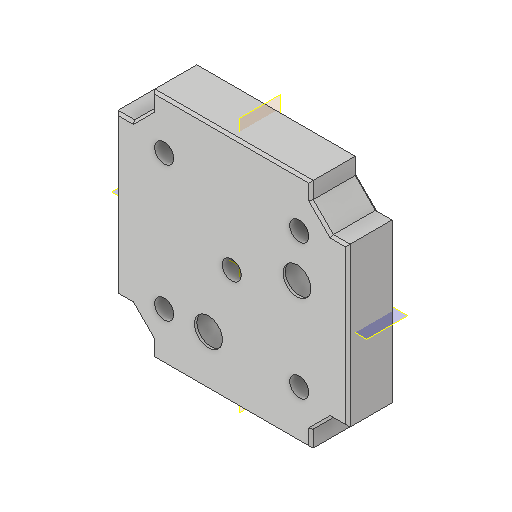
# Autodesk Inventor part: 20_Cube_Insert_Kinematic_Mirror_90_pro_magnetic
Saved by Autodesk Inventor 2022 (Build 260153000, 153)
## iProperties
Created: 2019-07-01
Part Number: 20_Cube_Insert_Kinematic_Mirror_90_pro_magnetic
Material: Generic
Document SubType Name: Modeling
Designer: diederichbenedict
Density: 1 g/cm^3
Appearance: Default
Catalog Web Link: isPrinted
Vendor: openUC2
Author: diederichbenedict
Autodesk Inventor part; units mm, degrees
ref_plane "YZ Plane" through (0, 0, 0) normal (1, 0, 0) x (0, 1, 0)
ref_plane "XZ Plane" through (0, 0, 0) normal (0, 1, 0) x (-1, 0, 0)
ref_plane "Work Plane1" through (0, 0, 10) normal (0, 0, 1) x (1, 0, 0)
sketch "Sketch1" plane through (0, 0, 10) normal (0, 0, 1) x (1, 0, 0)
  line L0 (-4.0299, -0.3538) -> (-2.2322, 1.4439) construction
  arc A0 (-1.4439, 2.2322) -> (-2.2322, 1.4439) centre (-0.9299, 0.9299) ccw construction
  line L1 (-1.4439, 2.2322) -> (0.3538, 4.0299) construction
  line L2 (-37.8299, 42.8299) -> (-37.8299, 37.8299) construction
  line L3 (-37.8299, 37.8299) -> (-42.9208, 37.8299) construction
  line L4 (-37.8299, 42.2137) -> (-37.8299, 45.8299) construction
  line L5 (-37.8299, 45.8299) -> (-4.0299, 45.8299) construction
  line L6 (-4.0299, 45.8299) -> (-4.0299, 42.2137) construction
  line L7 (-4.0299, 4.0299) -> (0.3538, 4.0299) projected
  circle A1 centre (-20.9299, 20.9299) radius 17.5 projected
  line L8 (-20.9299, 58.9723) -> (17.1124, 20.9299) construction
  line L9 (17.1124, 20.9299) -> (-20.9299, -17.1124) construction
  line L10 (-20.9299, -17.1124) -> (-58.9723, 20.9299) construction
  line L11 (-58.9723, 20.9299) -> (-20.9299, 58.9723) construction
  line L12 (-20.9299, 58.9723) -> (-20.9299, -17.1124) construction
  line L13 (17.1124, 20.9299) -> (-58.9723, 20.9299) construction
  line L14 (-20.9299, 58.9723) -> (32.8701, 58.9723) construction
  line L15 (-43.4299, 43.4299) -> (1.5701, 43.4299) construction
  line L16 (1.5701, 43.4299) -> (1.5701, -1.5701) construction
  line L17 (1.5701, -1.5701) -> (-43.4299, -1.5701) construction
  line L18 (-43.4299, -1.5701) -> (-43.4299, 43.4299) construction
  line L19 (-43.4299, 43.4299) -> (1.5701, -1.5701) construction
  line L20 (1.5701, 43.4299) -> (-43.4299, -1.5701) construction
  line L21 (-43.4299, 5.3876) -> (-43.4299, 36.4723)
  line L22 (-43.4299, 36.4723) -> (-36.4723, 43.4299)
  line L23 (-36.4723, 43.4299) -> (-5.3876, 43.4299)
  line L24 (-5.3876, 43.4299) -> (1.5701, 36.4723)
  line L25 (1.5701, 36.4723) -> (1.5701, 5.3876)
  line L26 (1.5701, 5.3876) -> (-5.3876, -1.5701)
  line L27 (-5.3876, -1.5701) -> (-36.4723, -1.5701)
  line L28 (-36.4723, -1.5701) -> (-43.4299, 5.3876)
  line L29 (-4.0299, 42.2137) -> (-37.8299, 42.2137) projected
  line L30 (-4.0299, -0.3538) -> (-4.0299, 4.0299) projected
  circle A2 centre (-20.9299, 20.9299) radius 1.5
  line L31 (-10.9299, 10.9299) -> (-30.9299, 10.9299) construction
  line L32 (-30.9299, 10.9299) -> (-30.9299, 30.9299) construction
  line L33 (-30.9299, 30.9299) -> (-10.9299, 30.9299) construction
  line L34 (-10.9299, 30.9299) -> (-10.9299, 10.9299) construction
  line L35 (-10.9299, 10.9299) -> (-30.9299, 30.9299) construction
  line L36 (-30.9299, 10.9299) -> (-10.9299, 30.9299) construction
  circle A3 centre (-30.9299, 30.9299) radius 1.4
  circle A4 centre (-30.9299, 10.9299) radius 1.4
  circle A5 centre (-10.9299, 10.9299) radius 1.4
  line L37 (-45.8299, 37.8299) -> (-42.0723, 37.8299) construction
  line L38 (-42.1723, 37.7299) -> (-45.8299, 37.7299)
  line L39 (-45.8299, 37.7299) -> (-45.8299, 4.1299)
  line L40 (-45.8299, 4.1299) -> (-42.1723, 4.1299)
  line L41 (-42.1723, 4.1299) -> (-42.1723, 37.7299)
  line L42 (-45.8299, 4.0299) -> (-42.0723, 4.0299) construction
  line L43 (-45.8299, 37.8299) -> (-42.0723, 37.8299) projected
  line L44 (-37.7299, 45.8299) -> (-4.1299, 45.8299)
  line L45 (-4.1299, 45.8299) -> (-4.1299, 42.1723)
  line L46 (-4.1299, 42.1723) -> (-37.7299, 42.1723)
  line L47 (-37.7299, 42.1723) -> (-37.7299, 45.8299)
  line L48 (0.4701, 37.8299) -> (0.4701, 4.0299) construction
  line L49 (0.4701, 4.0299) -> (3.9701, 4.0299) construction
  line L50 (3.9701, 37.8299) -> (3.9701, 4.0299) construction
  line L51 (0.4701, 37.8299) -> (3.9701, 37.8299) construction
  line L52 (-45.8299, -3.9701) -> (-4.0299, -3.9701) construction
  line L53 (0.3124, 37.7299) -> (3.9701, 37.7299)
  line L54 (3.9701, 37.7299) -> (3.9701, 4.1299)
  line L55 (3.9701, 4.1299) -> (0.3124, 4.1299)
  line L56 (0.3124, 4.1299) -> (0.3124, 37.7299)
  line L57 (-4.1713, -0.3538) -> (-37.7299, -0.3538)
  line L58 (-37.7299, -0.3538) -> (-37.7299, -3.9701)
  line L59 (-37.7299, -3.9701) -> (-4.1713, -3.9701)
  line L60 (-4.1713, -3.9701) -> (-4.1713, -0.3538)
  point P0 (-37.8299, 4.0299)
  dimension "d18" = 53.8
  dimension "d19" = 45
  dimension "d20" = 53.8
  dimension "d21" = 45
  dimension "d22" = 45
  dimension "d30" = 20
  dimension "d31" = 20
  dimension "d32" = 2.8
  dimension "d33" = 2.8
  dimension "d34" = 2.8
  dimension "d35" = 3
  dimension "d36" = 0.1
  dimension "d37" = 0.1
  dimension "d38" = 0.1
  dimension "d39" = 0.1
  constraints: 86 end point, 21 point on line, 14 parallel, 8 perpendicular, 7 horizontal, 7 midpoint, 4 centre point, 4 coincident, 1 equal length
  measures "d18" distance of L8.start L8.end
  measures "d19" angle of L8 L14
  measures "d20" distance of L8.end L9.end
  measures "d21" distance of L16.end L17.end
  measures "d22" distance of L15.end L16.end
  measures "d30" distance of L32.end L33.end
  measures "d31" distance of L31.end L32.end
  measures "d32" diameter of A3
  measures "d33" diameter of A4
  measures "d34" diameter of A5
  measures "d35" diameter of A2
  measures "d36" distance between parallel lines of L38 L43
  measures "d37" distance between parallel lines of L40 L42
  measures "d38" distance between parallel lines of L45 L6
  measures "d39" distance between parallel lines of L4 L47
extrude "Extrusion1" add sketch "Sketch1" along normal blind 10 contours L30 L26 L57 L28 L41 L22 L46 L24 L56 L7 | L7 L26 L30 | L56 L24 L25 L26 | L26 L25 L24 L53 L54 L55 | L60 L59 L58 L57 L28 L27 L26 | L26 L27 L28 L57 | L46 L22 L29 L24 | L24 L29 L45 | L40 L39 L38 L22 L21 L28 | L28 L21 L22 L41 | L29 L22 L23 L24 | L24 L23 L22 L29 L47 L44 L45 | L47 L29 L22 | A1 | A2 | A3 | A4 | A5
sketch "Skizze4" plane through (0, 0, 20) normal (0, 0, 1) x (1, 0, 0)
  line L0 (-37.7299, 42.1723) -> (-42.1723, 37.7299) projected
  line L1 (-42.1723, 37.7299) -> (-45.8299, 37.7299) projected
  line L2 (-45.8299, 37.7299) -> (-45.8299, 4.1299) construction
  line L3 (-45.8299, 4.1299) -> (-42.1723, 4.1299) projected
  line L4 (-42.1723, 4.1299) -> (-37.6885, -0.3538) projected
  line L5 (-37.6885, -0.3538) -> (-37.7299, -0.3538) projected
  line L6 (-37.7299, -0.3538) -> (-37.7299, -3.9701) projected
  line L7 (-37.7299, -3.9701) -> (-4.1713, -3.9701) construction
  line L8 (-4.1713, -3.9701) -> (-4.1713, -0.3538) projected
  line L9 (-4.1713, -0.3538) -> (0.3124, 4.1299) projected
  line L10 (0.3124, 4.1299) -> (3.9701, 4.1299) projected
  line L11 (3.9701, 4.1299) -> (3.9701, 37.7299) construction
  line L12 (3.9701, 37.7299) -> (0.3124, 37.7299) projected
  line L13 (0.3124, 37.7299) -> (-4.1299, 42.1723) projected
  line L14 (-4.1299, 42.1723) -> (-4.1299, 45.8299) projected
  line L15 (-4.1299, 45.8299) -> (-37.7299, 45.8299) construction
  line L16 (-37.7299, 45.8299) -> (-37.7299, 42.1723) projected
  line L17 (-37.9299, 46.0299) -> (-3.9299, 46.0299) construction
  line L18 (-3.9299, 46.0299) -> (-3.9299, 42.2551)
  line L19 (-3.9299, 42.2551) -> (0.3953, 37.9299)
  line L20 (0.3953, 37.9299) -> (4.1701, 37.9299)
  line L21 (4.1701, 37.9299) -> (4.1701, 3.9299) construction
  line L22 (4.1701, 3.9299) -> (0.3953, 3.9299)
  line L23 (0.3953, 3.9299) -> (-3.9713, -0.4367)
  line L24 (-3.9713, -0.4367) -> (-3.9713, -4.1701)
  line L25 (-3.9713, -4.1701) -> (-37.9299, -4.1701) construction
  line L26 (-37.9299, -4.1701) -> (-37.9299, -0.3953)
  line L27 (-37.9299, -0.3953) -> (-42.2551, 3.9299)
  line L28 (-42.2551, 3.9299) -> (-46.0299, 3.9299)
  line L29 (-46.0299, 3.9299) -> (-46.0299, 37.9299) construction
  line L30 (-46.0299, 37.9299) -> (-42.2551, 37.9299)
  line L31 (-42.2551, 37.9299) -> (-37.9299, 42.2551)
  line L32 (-37.9299, 42.2551) -> (-37.9299, 46.0299)
  line L33 (-45.8299, 37.7299) -> (-45.8299, 37.9299)
  line L34 (-4.1299, 45.8299) -> (-37.7299, 45.8299) projected
  line L35 (-37.7299, 45.8299) -> (-37.9299, 45.8299)
  line L36 (-4.1299, 45.8299) -> (-3.9299, 45.8299)
  line L37 (3.9701, 37.7299) -> (3.9701, 37.9299)
  line L38 (3.9701, 4.1299) -> (3.9701, 37.7299) projected
  line L39 (3.9701, 4.1299) -> (3.9701, 3.9299)
  line L40 (-4.1713, -3.9701) -> (-3.9713, -3.9701)
  line L41 (-37.7299, -3.9701) -> (-37.9299, -3.9701)
  line L42 (-45.8299, 4.1299) -> (-45.8299, 3.9299)
  point P0 (0, 0)
  dimension "d40" = 0.2
  constraints: 48 end point, 12 point on line, 4 perpendicular, 15 other
  measures "d40" distance between parallel lines of L15 L17
extrude "IM_offset" add sketch "Skizze4" against normal up to surface (10 mm away)
ref_plane "Work Plane5" through (-37.9299, 20.9299, 10) normal (0, -1, 0) x (1, 0, 0)
ref_plane "Work Plane6" through (-20.9299, 3.9299, 10) normal (1, 0, 0) x (0, 0, -1)
sketch "Sketch24" plane through (0, 0, 10) normal (0, 0, -1) x (-1, 0, 0)
  line L0 (6.4299, 6.4299) -> (35.4299, 6.4299) construction
  line L1 (35.4299, 6.4299) -> (35.4299, 35.4299) construction
  line L2 (35.4299, 35.4299) -> (6.4299, 35.4299) construction
  line L3 (6.4299, 35.4299) -> (6.4299, 6.4299) construction
  line L4 (6.4299, 6.4299) -> (35.4299, 35.4299) construction
  line L5 (35.4299, 6.4299) -> (6.4299, 35.4299) construction
  point P0 (0, 0)
  point P1 (20.9299, 20.9299)
  dimension "d143" = 29
  dimension "d144" = 29
  constraints: 12 end point, 2 midpoint, 2 parallel, 1 horizontal, 1 perpendicular
  measures "d143" distance of L2.end L1.end
  measures "d144" distance of L1.end L0.end
hole "Hole1" at (-20.9299, 20.9299, 10) at (-6.4299, 6.4299, 10) at (-35.4299, 6.4299, 10) at (-35.4299, 35.4299, 10) at (-6.4299, 35.4299, 10) direction (0, 0, 1) diameter 4.1 end through all
sketch "Skizze28" plane through (0, 0, 10) normal (0, 0, -1) x (-1, 0, 0)
  circle A0 centre (25.9299, 6.9299) radius 3 projected
  circle A1 centre (6.9299, 25.9299) radius 3 projected
  line L0 (9.9299, 4.9299) -> (1.9299, 4.9299) projected
  line L1 (4.9299, 1.9299) -> (1.9299, 4.9299) projected
  line L2 (36.9299, 1.9299) -> (4.9299, 1.9299) projected
  line L3 (39.9299, 4.9299) -> (36.9299, 1.9299) projected
  line L4 (39.9299, 36.9299) -> (39.9299, 4.9299) projected
  line L5 (36.9299, 39.9299) -> (39.9299, 36.9299) projected
  line L6 (4.9299, 39.9299) -> (36.9299, 39.9299) projected
  line L7 (1.9299, 36.9299) -> (4.9299, 39.9299) projected
  line L8 (1.9299, 8.9299) -> (1.9299, 36.9299) projected
  line L9 (1.9299, 8.9299) -> (9.9299, 8.9299) projected
  line L10 (9.9299, 8.9299) -> (9.9299, 4.9299) projected
  circle A2 centre (34.9299, 6.9299) radius 2 projected
  circle A3 centre (6.9299, 25.9299) radius 4.05
  circle A4 centre (25.9299, 6.9299) radius 4.05
  point P0 (0, 0)
  dimension "d173" = 8.1
  dimension "d174" = 8.1
  constraints: 2 centre point, 2 coincident
  measures "d173" diameter of A3
  measures "d174" diameter of A4
extrude "Extrusion23" cut sketch "Skizze28" against normal blind 9.5 contours A0 | A1 | A3 | A4
chamfer "Fase2" distance 0.5 angle 45 39 edges at (-2.8799, 25.9299, 10) (-6.4299, 33.3799, 10) (-20.9299, 18.8799, 10) (-6.4299, 4.3799, 10) (-21.8799, 6.9299, 10) (-35.4299, 33.3799, 10) (-35.4299, 4.3799, 10) (-45.8299, 20.9299, 10) (-40.0925, 1.7673, 10) (-44.0425, 3.9299, 10) (-37.9299, -2.1827, 10) (-20.9506, -3.9701, 10) (-3.9713, -2.2034, 10) (-1.788, 1.7466, 10) (3.9701, 20.9299, 20) (3.9701, 20.9299, 10) (2.1827, 3.9299, 10) (2.1827, 37.9299, 10) (-1.7673, 40.0925, 10) (-3.9299, 44.0425, 10) (-20.9299, 45.8299, 10) (-37.9299, 44.0425, 10) (-40.0925, 40.0925, 10) (-44.0425, 37.9299, 10) (-44.0425, 37.9299, 20) (-40.0925, 40.0925, 20) (-37.9299, 44.0425, 20) (-20.9299, 45.8299, 20) (-45.8299, 20.9299, 20) (-44.0425, 3.9299, 20) (-20.9506, -3.9701, 20) (-37.9299, -2.1827, 20) (-40.0925, 1.7673, 20) (-3.9713, -2.2034, 20) (-1.788, 1.7466, 20) (2.1827, 3.9299, 20) (2.1827, 37.9299, 20) (-1.7673, 40.0925, 20) (-3.9299, 44.0425, 20)
sketch "Skizze29" plane through (0, 0, 20) normal (0, 0, 1) x (1, 0, 0)
  circle A0 centre (-35.4299, 6.4299) radius 2.55 projected
  circle A1 centre (-25.9299, 6.9299) radius 4.55 projected
  circle A2 centre (-20.9299, 20.9299) radius 2.55 projected
  circle A3 centre (-6.9299, 25.9299) radius 4.55 projected
  circle A4 centre (-6.4299, 35.4299) radius 2.55 projected
  circle A5 centre (-6.4299, 6.4299) radius 2.55 projected
  circle A6 centre (-35.4299, 35.4299) radius 2.55 projected
  line L0 (3.4701, 4.4299) -> (3.4701, 37.4299) projected
  line L1 (0.1882, 4.4299) -> (3.4701, 4.4299) projected
  line L2 (-4.4713, -0.2296) -> (0.1882, 4.4299) projected
  line L3 (-4.4713, -3.4701) -> (-4.4713, -0.2296) projected
  line L4 (-37.4299, -3.4701) -> (-4.4713, -3.4701) projected
  line L5 (-37.4299, -0.1882) -> (-37.4299, -3.4701) projected
  line L6 (-42.048, 4.4299) -> (-37.4299, -0.1882) projected
  line L7 (-45.3299, 4.4299) -> (-42.048, 4.4299) projected
  line L8 (-45.3299, 37.4299) -> (-45.3299, 4.4299) projected
  line L9 (-42.048, 37.4299) -> (-45.3299, 37.4299) projected
  line L10 (-37.4299, 42.048) -> (-42.048, 37.4299) projected
  line L11 (-37.4299, 45.3299) -> (-37.4299, 42.048) projected
  line L12 (-4.4299, 45.3299) -> (-37.4299, 45.3299) projected
  line L13 (-4.4299, 42.048) -> (-4.4299, 45.3299) projected
  line L14 (0.1882, 37.4299) -> (-4.4299, 42.048) projected
  line L15 (3.4701, 37.4299) -> (0.1882, 37.4299) projected
  point P0 (0, 0)
hole "Bohrung2" at (-6.9299, 25.9299, 20) at (-25.9299, 6.9299, 20) direction (0, 0, -1) diameter 6 end through all
body "Solid1"
